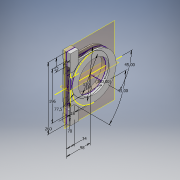
# Autodesk Inventor part: корпус п
Saved by Autodesk Inventor 2018.3 (Build 223284000, 284)
## iProperties
Created: 2018-05-23
Part Number: корпус п
Material: Типовые
Document SubType Name: Modeling
Designer: kriku
Density: 1 g/cm^3
Appearance: По умолчанию
Author: kriku
Autodesk Inventor part; units mm, degrees
ref_plane "XZ Plane" through (0, 0, 0) normal (0, 1, 0) x (-1, 0, 0)
sketch "Эскиз1" plane through (0, 0, 0) normal (1, 0, 0) x (0, 1, 0)
  circle A0 centre (0, 0) radius 65
  circle A1 centre (0, 0) radius 92.5
  line L0 (0, -92.5) -> (-64, -92.5)
  line L1 (-147.5584, 0) -> (132.5097, 0) projected
  line L2 (-64, -92.5) -> (-64, -130)
  line L3 (-64, -130) -> (-98, -130)
  line L4 (-64, 92.5) -> (-64, 130)
  line L5 (-64, 130) -> (-98, 130)
  line L6 (-98, 98) -> (-97, 98)
  line L7 (-97, 98) -> (-97, -98)
  line L8 (-97, -98) -> (-98, -98)
  line L9 (-98, 130) -> (-98, 98)
  line L10 (-98, -98) -> (-98, -130)
  line L11 (-64, -92.5) -> (-64, -78)
  line L12 (-64, -78) -> (-82, -60)
  line L13 (-82, -60) -> (-97, -60)
  line L14 (-64, 78) -> (-82, 60)
  line L15 (-82, 60) -> (-97, 60)
  line L16 (-64, 92.5) -> (-64, 78)
  line L17 (0, 92.5) -> (-64, 92.5)
  line L18 (-92.5, 0) -> (-97, 0)
  line L19 (65.4074, -65.4074) -> (0, 0)
  arc A2 (43.2175, -64.3311) -> (64.3311, -43.2175) centre (54.8008, -54.8008) ccw
  arc A3 (64.3311, 43.2175) -> (43.2175, 64.3311) centre (54.8008, 54.8008) ccw
  arc A4 (-43.2175, 64.3311) -> (-64.3311, 43.2175) centre (-54.8008, 54.8008) ccw
  arc A5 (-64.3311, -43.2175) -> (-43.2175, -64.3311) centre (-54.8008, -54.8008) ccw
  line L20 (-79.7385, 78) -> (-97, 78)
  line L21 (77.5, 0) -> (92.5, 0)
  line L22 (92.5, 0) -> (77.5, 0)
  line L23 (-77.5, 0) -> (-92.5, 0)
  arc A6 (64.3311, 43.2175) -> (43.2175, 64.3311) centre (54.8008, 54.8008) ccw
  arc A7 (-52.2768, 69.5869) -> (-64.3311, 43.2175) centre (-54.8008, 54.8008) ccw
  arc A8 (77.5, 0) -> (64.3311, 43.2175) centre (0, 0) ccw
  arc A9 (43.2175, 64.3311) -> (-43.2175, 64.3311) centre (0, 0) ccw
  arc A10 (-64.3311, 43.2175) -> (64.3311, -43.2175) centre (0, 0) ccw
  line L24 (-43.2175, 64.3311) -> (-60.1609, 74.1609)
  arc A11 (-64, 83.4262) -> (-60.1609, 74.1609) centre (-50.8999, 83.4262) ccw
  arc A12 (-79.7385, 78) -> (-64.3311, 43.2175) centre (-40.5268, 74.5657) ccw
  line L25 (-77.5, 0) -> (-97, 0)
  line L26 (0, 92.5) -> (-64, 92.5)
  line L27 (-64, 83.4262) -> (-64, 92.5)
  line L28 (-79.7385, 78) -> (-97, 78)
  line L29 (-97, 78) -> (-97, 0)
  arc A13 (-52.2768, 69.5869) -> (-64.3311, 43.2175) centre (-54.8008, 54.8008) ccw
  line L30 (0, 92.5) -> (-64, 92.5)
  line L31 (-64, 92.5) -> (-64, 83.4262)
  line L32 (-77.5, 0) -> (-97, 0)
  arc A14 (-64.3311, 43.2175) -> (-77.5, 0) centre (0, 0) ccw
  line L33 (-64.3311, 43.2175) -> (-97, 43.2175)
  line L34 (-97, 43.2175) -> (-97, 78)
  line L35 (-79.7385, 78) -> (-97, 78)
  point P0 (-79.3022, 47.6173)
  point P1 (-71.1456, 59.1147)
  dimension "d2" = 185
  dimension "d0" = 130
  dimension "d5" = 98
  dimension "d6" = 34
  dimension "d7" = 196
  dimension "d8" = 260
  dimension "d9" = 1
  dimension "d10" = 45
  dimension "d11" = 70
  dimension "d12" = 18
  dimension "d19" = 45
  dimension "d22" = 360
  dimension "d24" = 52
  dimension "d27" = 77.5
  constraints: 70 end point, 32 point on circle, 14 centre point, 14 perpendicular, 12 point on line, 8 coincident, 6 horizontal, 5 collinear, 5 symmetric about line, 4 vertical, 1 midpoint, 1 parallel, 1 tangent, 27 other
  measures "d0" diameter of A0
  measures "d5" distance from line of L10 point (0, 0)
  measures "d6" distance of L2.end L3.end
  measures "d7" distance of L6.end L7.end
  measures "d8" distance between parallel lines of L3 L5
  measures "d9" distance between parallel lines of L9 L7
  measures "d10" angle of L13 L12
  measures "d11" distance between parallel lines of L3 L13
  measures "d12" horizontal distance of L11.end L12.end
  measures "d19" angle of L1 L19
  measures "d24" distance between parallel lines of L20 L5
  measures "d27" radius of A10
extrude "Выдавливание1" add sketch "Эскиз1" along normal mid plane 32.5 contours L1 A1 A2 A10 L19 A0 | A0 L1 A10 A4 L24 A9 A3 A8 | A0 L19 A10 L1 | A8 A3 A1 L1 | A10 A5 A1 L1 | L1 A1 L33 A10 | A10 A2 L19 | L19 A2 A10 | A12 A1 A4 | L33 A1 A12 | A10 A5 | A1 A5 A10 A2 | A3 A9 A4 L24 A1 | A1 L24 A4 | A4 L24
extrude "Выдавливание2" add sketch "Эскиз1" along normal mid plane 31 contours L13 L12 L11 L2 L3 L10 L8 L7
mirror "Зеркальное отражение1" about plane through (0, 0, 0) normal (0, 0, 1) of "Выдавливание2"
extrude "Выдавливание3" add sketch "Эскиз1" along normal mid plane 32 contours A1 L0 L11 L12 L13 L7 L1
mirror "Зеркальное отражение2" about plane through (0, 0, 0) normal (0, 0, 1) of "Выдавливание3"
extrude "Выдавливание4" cut sketch "Эскиз1" along normal mid plane 20 contours A8 A3 A1 L1 | L1 A1 L33 A10 | L1 L7 L33 A1 | L33 A1 A12 | A3 A9 A4 L24 A1 | L33 L7 L15 L14 A12 A1 | A1 L24 A11 L16 L17 | L14 L15 L7 L20 A12
mirror "Зеркальное отражение3" about plane through (0, 0, 0) normal (0, 0, 1) of "Выдавливание4"
extrude "Выдавливание5" cut sketch "Эскиз1" along normal mid plane 25 contours L33 A1 A12 | L33 L7 L15 L14 A12 A1 | L14 L15 L7 L20 A12
mirror "Зеркальное отражение4" about plane through (0, 0, 0) normal (0, 0, 1) of "Выдавливание5"
sketch "Эскиз2" plane through (16, 0, 0) normal (1, 0, 0) x (0, 0, -1)
  line L0 (-43.2175, -64.3311) -> (-43.2175, -97) projected
  arc A0 (-92.5, 0) -> (92.5, 0) centre (0, 0) ccw projected
  arc A1 (-43.2175, -81.7832) -> (0, -92.5) centre (0, 0) ccw
  line L1 (0, -92.5) -> (0, -97)
  line L2 (60, -97) -> (-60, -97) projected
  line L3 (0, -97) -> (-43.2175, -97)
  constraints: 4 end point, 4 point on circle, 1 centre point, 1 coincident, 1 collinear, 1 midpoint, 1 point on line
